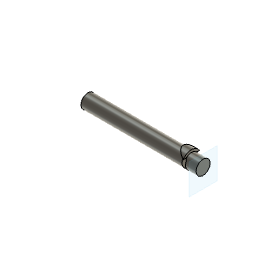
Handheld pitch slider v11 (Autodesk Fusion 360 archive; units mm, degrees)
design "whistle-pipe"
Autodesk Fusion 360 part; units mm, degrees
sketch "Sketch1" plane through (0, 0, 0) normal (0, 1, 0) x (1, 0, 0) in component "whistle v2"
  line L0 (15, 15) -> (-15, 15)
  line L1 (-15, 15) -> (-15, -15)
  line L2 (-15, -15) -> (15, -15)
  line L3 (15, -15) -> (15, 15)
  line L4 (15, 15) -> (-15, -15) construction
  line L5 (-15, 15) -> (15, -15) construction
  dimension "d1" = 30
  dimension "d2" = 30
  constraint horizontal L0
  constraint perpendicular L0 L1
  constraint parallel L0 L2
  constraint parallel L1 L3
  constraint coincident L4 origin
  constraint coincident L5 origin
  measures "d1" distance of L1.end L2.end
  measures "d2" distance of L0.end L1.end
extrude "Extrude1" add sketch "Sketch1" against normal blind 8 makes body 1 in component "whistle v2"
sketch "Sketch2" plane through (15, 0, 0) normal (1, 0, 0) x (0, 0, -1) in component "whistle v2"
  line L0 (15, -8) -> (15, 0)
  line L1 (-15, -8) -> (15, -8)
  line L2 (-15, 0) -> (-15, -8)
  line L3 (15, 0) -> (-15, 0)
  circle A0 centre (0, 0) radius 3
  circle A1 centre (0, 0) radius 4
  dimension "d22" = 6
  dimension "d24" = 8
  constraint coincident A0.centre A1.centre
  constraint concentric A0 A1
  measures "d22" diameter of A0
  measures "d24" diameter of A1
extrude "Extrude2" add sketch "Sketch2" against normal blind 30 contours L3 A0 A1 picked at (-3.6406, 0.3478) bodies 1 in component "whistle v2"
sketch "Sketch3" plane through (0, 0, 0) normal (0, 0, 1) x (1, 0, 0) in component "whistle v2"
  line L0 (10, 2) -> (1.5494, 6.8789)
  line L1 (10, 2) -> (20.2575, 2) construction
  line L2 (1.5494, 6.8789) -> (10, 6.8789)
  line L3 (10, 6.8789) -> (10, 2)
  dimension "d9" = 150
  constraint horizontal L1
  constraint horizontal L2
  constraint perpendicular L2 L3
  measures "d9" angle of L0 L1
extrude "Extrude5" cut sketch "Sketch2" against normal blind 30 contours L3 A0 picked at (-0.7331, -0.6802) bodies 1 in component "whistle v2"
sketch "Sketch5" plane through (-15, 0, 0) normal (-1, 0, 0) x (0, 0, 1) in component "whistle v2"
  circle A0 centre (0, 0) radius 3
  arc A1 (4, 0) -> (-4, 0) centre (0, 0) ccw
  line L0 (-4, 0) -> (-15, 0)
  line L1 (-15, 0) -> (-15, -8)
  line L2 (-15, -8) -> (15, -8)
  line L3 (15, -8) -> (15, 0)
  line L4 (15, 0) -> (4, 0)
  circle A2 centre (0, 0) radius 4
  constraint coincident A0.centre A1.centre
extrude "Extrude6" add sketch "Sketch5" against normal blind 5 contours A0 | A1 A2 bodies 1 in component "whistle v2"
extrude "Extrude3" cut sketch "Sketch3" along normal through all and the other way through all bodies 1 in component "whistle v2"
sketch "Sketch4" plane through (10, 0, 0) normal (-1, 0, 0) x (0, 0, 1) in component "whistle v2"
  arc A0 (3.4641, 2) -> (-3.4641, 2) centre (0, 0) ccw
  line L0 (-3.4641, 2) -> (-2.2361, 2)
  arc A1 (2.2361, 2) -> (-2.2361, 2) centre (0, 0) ccw
  line L1 (2.2361, 2) -> (3.4641, 2)
  line L2 (-3.4641, 2) -> (3.4641, 2)
  line L3 (3.4641, 2) -> (3.4641, -4.5612)
  line L4 (3.4641, -4.5612) -> (-3.4641, -4.5612)
  line L5 (-3.4641, -4.5612) -> (-3.4641, 2)
  circle A2 centre (0, 0) radius 4
  dimension "d23" = 8
  constraint horizontal L2
  constraint vertical L3
  constraint horizontal L4
  constraint vertical L5
  constraint coincident A0.end L0.start
  constraint coincident A0.start L1.end
  measures "d23" diameter of A2
extrude "Extrude4" add sketch "Sketch4" along normal blind 1 and the other way blind 0.5 contours L0 L1 L2 L3 L5 A2 | L3 L4 L5 A2 bodies 1 in component "whistle v2"
fillet "Fillet1" radius 1 2 edges at (9, 2, 0) (10.5, 2, 0) on bodies 1 in component "whistle v2"
extrude "Extrude7" cut 1 faces at (5, 0, -7.6667) along direction (0, -1, 0) blind 5 on bodies 1 bodies 1 in component "whistle v2"
extrude "Extrude8" cut 1 faces at (5, 0, 11.3333) along direction (0, -1, 0) blind 8 on bodies 1 bodies 1 in component "whistle v2"
extrude "Extrude9" add 1 faces at (-15, -4.3333, 1.3333) along direction (-1, 0, 0) blind 62.2231 on bodies 1 bodies 1 in component "whistle v2"
extrude "Extrude10" cut 1 faces at (-10, 1.0214, -1.0659) along direction (-1, 0, 0) blind 62.2231 on bodies 1 bodies 1 in component "whistle v2"
extrude "Extrude11" add 1 faces at (-72.2231, 0.8292, -0.2558) along direction (1, 0, 0) blind 8.8618 on bodies 1 bodies 1 in component "whistle v2"
extrude "Extrude12" cut 1 faces at (-77.2231, -4.3333, 1.3333) along direction (1, 0, 0) blind 8.8618 on bodies 1 bodies 1 in component "whistle v2"
extrude "Extrude13" add 1 faces at (-63.3614, 0.8292, -0.2558) along direction (1, 0, 0) blind 7.8947 on bodies 1 bodies 1 in component "whistle v2"
extrude "Extrude14" cut 1 faces at (-68.3614, -4.3333, 1.3333) along direction (1, 0, 0) blind 7.8947 on bodies 1 bodies 1 in component "whistle v2"
extrude "Extrude15" add 1 faces at (-55.4667, 1.0214, -1.0659) along direction (1, 0, 0) blind 3.6181 on bodies 1 bodies 1 in component "whistle v2"
extrude "Extrude16" cut 1 faces at (-60.4667, -4.3333, 1.3333) along direction (1, 0, 0) blind 3.6181 on bodies 1 bodies 1 in component "whistle v2"
extrude "Extrude17" add 1 faces at (-51.8486, 1.0214, -1.0659) along direction (1, 0, 0) blind 6.6387 on bodies 1 bodies 1 in component "whistle v2"
extrude "Extrude18" cut 1 faces at (-56.8486, -4.3333, 1.3333) along direction (1, 0, 0) blind 6.6387 on bodies 1 bodies 1 in component "whistle v2"
extrude "Extrude19" add 1 faces at (-45.2099, 1.0214, -1.0659) along direction (1, 0, 0) blind 5.9144 on bodies 1 bodies 1 in component "whistle v2"
extrude "Extrude20" cut 1 faces at (-50.2099, -4.3333, 1.3333) along direction (1, 0, 0) blind 5.9144 on bodies 1 bodies 1 in component "whistle v2"
extrude "Extrude21" add 1 faces at (-39.2955, 1.0214, -1.0659) along direction (1, 0, 0) blind 5.269 on bodies 1 bodies 1 in component "whistle v2"
extrude "Extrude22" cut 1 faces at (-44.2955, -4.3333, 1.3333) along direction (1, 0, 0) blind 5.269 on bodies 1 bodies 1 in component "whistle v2"
move_body "Move1" bodies 1 to x (1, 0, 0) y (0, 0, 1) z (0, -1, 0) at (0, -4, 12) in component "whistle v2"
move_face "OffsetFaces1" offset -9 1 faces at (-21.0176, 11, 6) on bodies 1 in component "whistle v2"
sketch "Sketch1 (2)" plane through (15, 0, 0) normal (1, 0, 0) x (0, 1, 0)
  line L0 (-8, 12) -> (-8, 4)
  line L1 (-8, 4) -> (2, 4)
  line L2 (2, 4) -> (2, 7)
  line L3 (2, 7) -> (0, 7)
  line L4 (0, 7) -> (0, 12)
  line L5 (-9.9872, 4) -> (2, 4)
  line L6 (2, 4) -> (2, 17)
  line L7 (2, 17) -> (-9.9872, 17)
  line L8 (-9.9872, 17) -> (-9.9872, 4)
  circle A0 centre (-4, 12) radius 3
  arc A1 (0, 12) -> (-8, 12) centre (-4, 12) ccw
  circle A2 centre (-4, 12) radius 3
  dimension "d62" = 6
  constraint horizontal L5
  constraint vertical L6
  constraint horizontal L7
  constraint vertical L8
  measures "d62" diameter of A0
extrude "Extrude23" add sketch "Sketch1 (2)" against normal blind 3 contours L0 L1 L2 L3 L4 L5 L6 A1 | L0 L3 L4 L5 L6 L7 L8 A1 | A0 A2 bodies 1 in component "whistle v2"
sketch "Sketch2 (2)" plane through (15, 0, 0) normal (1, 0, 0) x (0, 1, 0)
  line L0 (-9.9872, 4) -> (2, 4)
  line L1 (2, 4) -> (2, 17)
  line L2 (2, 17) -> (-9.9872, 17)
  line L3 (-9.9872, 17) -> (-9.9872, 4)
hole "Hole1" at (15, -4, 12) direction (-1, 0, 0) diameter 6 depth 3 tip angle 180 bodies 1 in component "whistle v2"
extrude "Extrude24" cut 1 faces at (-22.0176, 0.6667, 7) along direction (0, 0, -1) blind 3 on bodies 1 bodies 1 in component "whistle v2"
extrude "Extrude25" cut 2 faces at (12, 0.6667, 6) (12, -9.3248, 11) along direction (1, 0, 0) blind 3 on bodies 1 bodies 1 in component "whistle v2"
sketch "Sketch3 (2)" plane through (-39.0264, 0, 0) normal (-1, 0, 0) x (0, -1, 0)
  line L0 (0, 12) -> (0, 4)
  line L1 (0, 4) -> (8, 4)
  line L2 (8, 4) -> (8, 12)
  arc A0 (8, 12) -> (0, 12) centre (4, 12) ccw
extrude "Extrude1'" add sketch "Sketch3 (2)" against normal blind 54.026 separate body makes body 2
combine "Combine1" operation cut target body 2 tool bodies 1
component "whistle v2" placed x (1, 0, 0) y (0, 1, 0) z (0, 0, 1) at (0, 0, 0)
equation "tube_length = 20 mm"
equation "d19 = -25 mm + tube_length"
equation "d27 = 81.2231247 mm - 19 mm"
equation "d29 = -81.2231247 mm + 19 mm"
